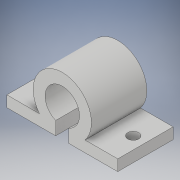
# Autodesk Inventor part: motor_cover_part2
Saved by Autodesk Inventor 2019 (Build 230136000, 136)
## iProperties
Created: 2019-08-13
Part Number: motor_cover_part2
Material: 一般
Document SubType Name: Modeling
Designer: naito
Density: 1 g/cm^3
Appearance: 既定
Author: naito
Autodesk Inventor part; units mm, degrees
ref_plane "YZ Plane" through (0, 0, 0) normal (1, 0, 0) x (0, 1, 0)
ref_plane "XZ Plane" through (0, 0, 0) normal (0, 1, 0) x (-1, 0, 0)
ref_plane "XY Plane" through (0, 0, 0) normal (0, 0, 1) x (1, 0, 0)
sketch "スケッチ1" plane through (0, 0, 0) normal (0, 0, 1) x (1, 0, 0)
  arc A0 (1.1923, -2.8615) -> (-1.1923, -2.8615) centre (0, 0) ccw
  arc A1 (4.1155, -3.2597) -> (-4.1155, -3.2597) centre (0, 0) ccw
  line L0 (-10, -3.2597) -> (-4.1155, -3.2597)
  line L1 (10, -3.2597) -> (10, -5.2597)
  line L2 (10, -5.2597) -> (1.1923, -5.2597)
  line L3 (-10, -5.2597) -> (-10, -3.2597)
  line L4 (4.1155, -3.2597) -> (10, -3.2597)
  line L5 (1.1923, -5.2597) -> (1.1923, -2.8615)
  line L6 (-1.1923, -2.8615) -> (-1.1923, -5.2597)
  line L7 (-1.1923, -5.2597) -> (-10, -5.2597)
  dimension "d0" = 6.2
  dimension "d1" = 10.5
  dimension "d2" = 20
  dimension "d5" = 2
  constraints: 16 end point, 6 parallel, 4 point on circle, 2 centre point, 2 coincident, 2 horizontal, 2 perpendicular, 1 collinear
  measures "d0" diameter of A0
  measures "d1" diameter of A1
  measures "d2" distance of L1.end L3.start
  measures "d5" distance between parallel lines of L2 L4
extrude "押し出し1" add sketch "スケッチ1" along normal blind 10
sketch "スケッチ2" plane through (-10, -3.2597, 0) normal (0, 1, 0) x (1, 0, 0)
  circle A0 centre (2.2, -5) radius 1
  circle A1 centre (17.8, -5) radius 1
  line L0 (0, 0) -> (0, -10) projected
  point P0 (10, 0)
  point P1 (0, -5)
  dimension "d8" = 2
  dimension "d9" = 2
  dimension "d10" = 15.6
  dimension "d11" = 2.2
  constraints: 2 centre point, 2 horizontal alignment, 1 midpoint
  measures "d8" diameter of A0
  measures "d9" diameter of A1
  measures "d10" distance of A1.centre A0.centre
  measures "d11" distance from line of A0.centre L0
extrude "押し出し2" cut sketch "スケッチ2" against normal blind 10
